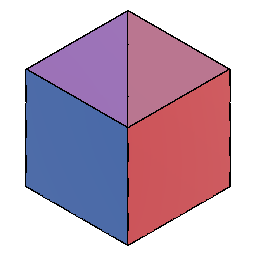
arena_QSCR (Autodesk Fusion 360 archive; units mm, degrees)
design "box_50x50x50cm"
Autodesk Fusion 360 part; units mm, degrees
sketch "Sketch7" plane through (0, 0, 0) normal (0, 1, 0) x (1, 0, 0)
  line L0 (253, -253) -> (-253, -253)
  line L1 (-253, -253) -> (-253, 253)
  line L2 (-253, 253) -> (253, 253)
  line L3 (253, 253) -> (253, -253)
  line L4 (253, -253) -> (-253, 253) construction
  line L5 (-253, -253) -> (253, 253) construction
  line L6 (250, 37.5) -> (253, 37.5)
  line L7 (253, 37.5) -> (253, -37.5)
  line L8 (253, -37.5) -> (250, -37.5)
  line L9 (250, -37.5) -> (250, 37.5)
  line L10 (-300, 0) -> (300, 0) construction
  line L11 (253, -112.5) -> (253, -187.5)
  line L12 (250, -112.5) -> (253, -112.5)
  line L13 (250, -187.5) -> (250, -112.5)
  line L14 (253, -187.5) -> (250, -187.5)
  line L15 (253, 187.5) -> (253, 112.5)
  line L16 (250, 187.5) -> (253, 187.5)
  line L17 (250, 112.5) -> (250, 187.5)
  line L18 (253, 112.5) -> (250, 112.5)
  line L19 (187.5, 253) -> (187.5, 250)
  line L20 (-112.5, 250) -> (-187.5, 250)
  line L21 (-187.5, 250) -> (-187.5, 253)
  line L22 (112.5, 253) -> (187.5, 253)
  line L23 (187.5, 250) -> (112.5, 250)
  line L24 (37.5, 250) -> (-37.5, 250)
  line L25 (-37.5, 250) -> (-37.5, 253)
  line L26 (-37.5, 253) -> (37.5, 253)
  line L27 (-112.5, 253) -> (-112.5, 250)
  line L28 (0, -300) -> (0, 300) construction
  line L29 (37.5, 253) -> (37.5, 250)
  line L30 (112.5, 250) -> (112.5, 253)
  line L31 (-187.5, 253) -> (-112.5, 253)
  line L32 (-253, 187.5) -> (-250, 187.5)
  line L33 (-250, -112.5) -> (-250, -187.5)
  line L34 (-250, -187.5) -> (-253, -187.5)
  line L35 (-253, 112.5) -> (-253, 187.5)
  line L36 (-250, 187.5) -> (-250, 112.5)
  line L37 (-250, 37.5) -> (-250, -37.5)
  line L38 (-250, -37.5) -> (-253, -37.5)
  line L39 (-253, -37.5) -> (-253, 37.5)
  line L40 (-253, -112.5) -> (-250, -112.5)
  line L41 (300, 0) -> (-300, 0) construction
  line L42 (-253, 37.5) -> (-250, 37.5)
  line L43 (-250, 112.5) -> (-253, 112.5)
  line L44 (-253, -187.5) -> (-253, -112.5)
  line L45 (-187.5, -253) -> (-187.5, -250)
  line L46 (112.5, -250) -> (187.5, -250)
  line L47 (187.5, -250) -> (187.5, -253)
  line L48 (-112.5, -253) -> (-187.5, -253)
  line L49 (-187.5, -250) -> (-112.5, -250)
  line L50 (-37.5, -250) -> (37.5, -250)
  line L51 (37.5, -250) -> (37.5, -253)
  line L52 (37.5, -253) -> (-37.5, -253)
  line L53 (112.5, -253) -> (112.5, -250)
  line L54 (0, 300) -> (0, -300) construction
  line L55 (-37.5, -253) -> (-37.5, -250)
  line L56 (-112.5, -250) -> (-112.5, -253)
  line L57 (187.5, -253) -> (112.5, -253)
  dimension "d15" = 506
  dimension "d16" = 506
  dimension "d17" = 3
  dimension "d18" = 75
  dimension "d21" = 0
  dimension "d22" = 150
  dimension "d24" = 360
  constraint horizontal L0
  constraint perpendicular L0 L1
  constraint parallel L0 L2
  constraint parallel L1 L3
  constraint coincident L4 origin
  constraint coincident L5 origin
  constraint horizontal L6
  constraint vertical L7
  constraint horizontal L8
  constraint vertical L9
  constraint collinear L3 L7
  constraint perpendicular L3 L10
  constraint symmetric L6 L8 L10
  measures "d15" distance of L1.end L2.end
  measures "d16" distance of L0.end L1.end
  measures "d17" distance of L6.start L6.end
  measures "d18" distance of L6.start L8.end
extrude "Extrude7" add sketch "Sketch7" along normal blind 3 contours L0 L1 L2 L3 L6 L8 L9 L12 L13 L14 L16 L17 L18 L19 L20 L21 L23 L24 L25 L27 L29 L30 L32 L33 L34 L36 L37 L38 L40 L42 L43 L45 L46 L47 L49 L50 L51 L53 L55 L56 makes body 1
sketch "Sketch9" plane through (0, 0, 253) normal (0, 0, 1) x (1, 0, 0)
  line L0 (-253, 0) -> (-187.5, 0)
  line L1 (-187.5, 0) -> (-187.5, 3)
  line L2 (-187.5, 3) -> (-253, 3)
  line L3 (-253, 3) -> (-253, 0)
  line L4 (-253, 0) -> (253, 0)
  line L5 (253, 0) -> (253, 506)
  line L6 (253, 506) -> (-253, 506)
  line L7 (-253, 506) -> (-253, 0)
  line L8 (-253, 287.5) -> (-250, 287.5)
  line L9 (-250, 287.5) -> (-250, 212.5)
  line L10 (-250, 212.5) -> (-253, 212.5)
  line L11 (-253, 212.5) -> (-253, 287.5)
  line L12 (-500, 250) -> (500, 250) construction
  line L13 (-253, 62.5) -> (-253, 137.5)
  line L14 (-253, 137.5) -> (-250, 137.5)
  line L15 (-250, 137.5) -> (-250, 62.5)
  line L16 (-250, 62.5) -> (-253, 62.5)
  line L17 (-253, 362.5) -> (-253, 437.5)
  line L18 (-253, 437.5) -> (-250, 437.5)
  line L19 (-250, 437.5) -> (-250, 362.5)
  line L20 (-250, 362.5) -> (-253, 362.5)
  dimension "d27" = 506
  dimension "d28" = 506
  dimension "d29" = 3
  dimension "d30" = 75
  dimension "d33" = 0
  dimension "d34" = 150
  constraint horizontal L4
  constraint vertical L5
  constraint horizontal L6
  constraint vertical L7
  constraint coincident L0.start L3.end
  constraint horizontal L8
  constraint vertical L9
  constraint horizontal L10
  constraint vertical L11
  constraint collinear L7 L11
  constraint perpendicular L5 L12
  constraint symmetric L8 L10 L12
  measures "d27" distance of L0.start L4.end
  measures "d28" distance of L0.start L6.end
  measures "d29" distance of L8.start L8.end
  measures "d30" distance of L8.start L10.end
extrude "Extrude8" add sketch "Sketch9" against normal blind 3 separate body contours L1 L2 L4 L5 L6 L7 L8 L9 L10 L14 L15 L16 L18 L19 L20 makes body 2
combine "Combine1" operation cut target body 2 tool bodies 1 keep tools
pattern_circular "C-Pattern1" count 2 over 90 about axis through (0, 1.75, 0) along (0, 1, 0) of bodies 2 makes body 3
combine "Combine2" operation cut target body 2 tool bodies 3
move_face "OffsetFaces1" offset -0.4 12 faces at (252, 437.5, 252) (252, 287.5, 252) (252, 137.5, 252) (252, 362.5, 251) (252, 212.5, 251) (252, 62.5, 251) (187.5, 1, 251) (37.5, 2, 251) (-112.5, 1, 251) (-187.5, 1, 252) (-37.5, 1, 252) (112.5, 1, 252) on bodies 2
pattern_circular "C-Pattern2" count 4 over 360 about axis through (0, 1.75, 0) along (0, 1, 0) of bodies 2 makes body 4 at (253, 192.5333, 12.3667) makes body 5 at (12.3667, 192.5333, -253) makes body 6 at (-253, 192.5333, -12.3667)
copy_body "Body->Comp1" bodies 1 removing the originals makes body 7 in component "Component"
copy_body "Body->Comp2" bodies 2 removing the originals makes body 8 in component "Component'"
copy_body "Body->Comp3" bodies 4 removing the originals makes body 9 in component "Component''"
copy_body "Body->Comp4" bodies 6 removing the originals makes body 10 in component "Component'''"
copy_body "Body->Comp5" bodies 5 removing the originals makes body 11 in component "Component''''"
component "Component" placed x (1, 0, 0) y (0, 1, 0) z (0, 0, 1) at (0, 0, 0)
component "Component'" placed x (1, 0, 0) y (0, 1, 0) z (0, 0, 1) at (0, 0, 0)
component "Component''" placed x (1, 0, 0) y (0, 1, 0) z (0, 0, 1) at (0, 0, 0)
component "Component'''" placed x (1, 0, 0) y (0, 1, 0) z (0, 0, 1) at (0, 0, 0)
component "Component''''" placed x (1, 0, 0) y (0, 1, 0) z (0, 0, 1) at (0, 0, 0)
equation "width = 500 mm"
equation "thick = 3 mm"
equation "d15 = width + thick * 2"
equation "d16 = width + thick * 2"
equation "d17 = thick"
equation "d27 = width + thick * 2"
equation "d28 = width + thick * 2"
equation "d29 = thick"
equation "offset = -0.4 mm"
equation "d40 = offset"
